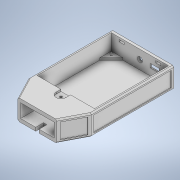
# Autodesk Inventor part: Bottom
Saved by Autodesk Inventor 2021 (Build 250183000, 183)
## iProperties
Created: 2021-04-28
Part Number: Bottom
Material: Generic
Document SubType Name: Modeling
Designer: mista
Density: 1 g/cm^3
Appearance: Default
Author: mista
Autodesk Inventor part; units mm, degrees
ref_plane "YZ Plane" through (0, 0, 0) normal (1, 0, 0) x (0, 1, 0)
ref_plane "XZ Plane" through (0, 0, 0) normal (0, 1, 0) x (-1, 0, 0)
ref_plane "XY Plane" through (0, 0, 0) normal (0, 0, 1) x (1, 0, 0)
sketch "Sketch1" plane through (0, 0, 0) normal (0, 1, 0) x (-1, 0, 0)
  line L0 (0, 0) -> (54.0004, 0)
  line L1 (54.0004, 0) -> (54.0004, -70.6374)
  line L2 (54.0004, -70.6374) -> (0, -70.6374)
  line L3 (0, -70.6374) -> (0, 0)
  circle A0 centre (51.9049, -68.5419) radius 1.0795
  circle A1 centre (3.3909, -67.8053) radius 1.0795
  circle A2 centre (51.9049, -1.8923) radius 1.0795
  circle A3 centre (1.7674, -2.3495) radius 1.0795
  dimension "d0" = 54.0004
  dimension "d1" = 70.6374
  dimension "d2" = 2.159
  dimension "d6" = 1.016
  dimension "d8" = 1.016
  dimension "d11" = 2.159
  dimension "d12" = 48.514
  dimension "d13" = 1.7526
  dimension "d15" = 66.6496
  dimension "d16" = 2.159
  dimension "d17" = 1.016
  dimension "d18" = 2.159
  dimension "d20" = 65.4558
  dimension "d21" = 50.1375
  constraints: 8 end point, 4 centre point, 2 parallel, 1 horizontal, 1 perpendicular
  measures "d0" distance of L1.end L2.end
  measures "d1" distance of L0.end L1.end
  measures "d2" diameter of A0
  measures "d6" distance edge to line of A0 L2
  measures "d8" distance edge to line of A0 L1
  measures "d11" diameter of A1
  measures "d12" horizontal distance of A1.centre A0.centre
  measures "d13" distance edge to line of A1 L2
  measures "d15" distance of A0.centre A2.centre
  measures "d16" diameter of A2
  measures "d17" distance edge to line of A2 L1
  measures "d18" diameter of A3
  measures "d20" vertical distance of A1.centre A3.centre
  measures "d21" horizontal distance of A3.centre A2.centre
sketch "Sketch2" plane through (0, 0, 0) normal (0, 1, 0) x (-1, 0, 0)
  line L0 (54.0004, 0) -> (54.0004, -70.6374) projected
  line L1 (0, 0) -> (54.0004, 0) projected
  line L2 (0, -70.6374) -> (0, 0) projected
  line L3 (54.0004, -70.6374) -> (0, -70.6374) projected
  line L4 (55.2704, -71.9074) -> (55.2704, 1.27)
  line L5 (55.2704, 1.27) -> (-1.27, 1.27)
  line L6 (-1.27, 1.27) -> (-1.27, -71.9074)
  line L7 (-1.27, -71.9074) -> (55.2704, -71.9074)
  line L8 (57.8104, 3.81) -> (57.8104, -74.4474)
  line L9 (57.8104, -74.4474) -> (-3.81, -74.4474)
  line L10 (-3.81, -74.4474) -> (-3.81, 3.81)
  line L11 (-3.81, 3.81) -> (57.8104, 3.81)
  dimension "d22" = 1.27
  dimension "d23" = 2.54
  constraints: 16 end point, 6 other
  measures "d22" distance between parallel lines of L0 L4
  measures "d23" distance between parallel lines of L4 L8
extrude "Extrusion1" add sketch "Sketch2" against normal blind 2.54 contours L0 L3 L2 L1 | L7 L6 L5 L4 | L8 L9 L10 L11
extrude "Extrusion2" add sketch "Sketch2" along normal blind 15.24 contours L8 L9 L10 L11
sketch "Sketch3" plane through (0, 0, 0) normal (0, 1, 0) x (1, 0, 0)
  line L0 (-55.2704, 71.9074) -> (-55.2704, -1.27) projected
  line L1 (-55.2704, -1.27) -> (1.27, -1.27) projected
  line L2 (1.27, -1.27) -> (1.27, 71.9074) projected
  line L3 (1.27, 71.9074) -> (-55.2704, 71.9074) projected
  line L4 (1.27, 10.16) -> (-10.16, -1.27)
  line L5 (-0.6357, 8.2543) -> (6.4192, 8.2543) construction
  line L6 (1.27, -1.27) -> (-55.2704, -1.27) construction
  line L7 (-27.0002, -1.27) -> (-27.0002, 8.9046) construction
  line L8 (1.27, 71.9074) -> (1.27, -1.27) construction
  line L9 (1.27, 35.3187) -> (-18.2366, 35.3187) construction
  line L10 (-55.2704, 10.16) -> (-43.8404, -1.27)
  line L11 (1.27, 60.4774) -> (-10.16, 71.9074)
  line L12 (-55.2704, 60.4774) -> (-43.8404, 71.9074)
  point P0 (0, 0)
  point P1 (-10.16, 71.9074)
  point P2 (1.27, 60.4774)
  point P3 (-55.2704, 60.4774)
  point P4 (-43.8404, 71.9074)
  dimension "d28" = 135
  dimension "d29" = 11.43
  constraints: 14 end point, 6 symmetric about line, 3 point on line, 2 horizontal, 2 midpoint, 1 vertical
  measures "d28" angle of L4 L5
  measures "d29" horizontal distance of L4.start L4.end
extrude "Extrusion3" add sketch "Sketch3" along normal blind 2.032 contours L3 L12 L0 | L10 L1 L0 | L3 L2 L11 | L4 L2 L1
extrude "Extrusion4" add sketch "Sketch1" along normal blind 3.81 contours A0 | A1 | A2 | A3
thicken "Thicken1" operation add thickness 0.127 both sides no extend neighbours yes toward (0.8451901, 0, -0.5344658) faces at (-4.3033, 3.2173, -67.2283)
thicken "Thicken2" operation add thickness 0.127 both sides no extend neighbours yes toward (0.9870503, 0, -0.1604113) faces at (-2.8329, 3.2173, -2.1763)
thicken "Thicken3" operation add thickness 0.127 both sides no extend neighbours yes toward (-0.6324454, 0, -0.774605) faces at (-51.2222, 3.2173, -1.0561)
thicken "Thicken4" operation add thickness 0.127 both sides no extend neighbours yes toward (-0.8451901, 0, 0.5344658) faces at (-50.9925, 2.6247, -69.1189)
sketch "Sketch10" plane through (3.81, -2.54, -74.4474) normal (0, 0, -1) x (-1, 0, 0)
  line L0 (20.6248, 13.4112) -> (20.6248, 9.6012)
  line L1 (20.6248, 9.6012) -> (11.7348, 9.6012)
  line L2 (11.7348, 9.6012) -> (11.7348, 13.4112)
  line L3 (11.7348, 13.4112) -> (20.6248, 13.4112)
  line L4 (0, 0) -> (0, 17.78)
  line L5 (61.6204, 0) -> (0, 0)
  line L6 (61.6204, 17.78) -> (61.6204, 0)
  line L7 (0, 17.78) -> (61.6204, 17.78)
  line L8 (22.1488, 13.9192) -> (22.1488, 9.0932)
  line L9 (21.1328, 8.0772) -> (11.2268, 8.0772)
  line L10 (10.2108, 9.0932) -> (10.2108, 13.9192)
  line L11 (11.2268, 14.9352) -> (21.1328, 14.9352)
  arc A0 (11.2268, 14.9352) -> (10.2108, 13.9192) centre (11.2268, 13.9192) ccw
  arc A1 (22.1488, 13.9192) -> (21.1328, 14.9352) centre (21.1328, 13.9192) ccw
  arc A2 (21.1328, 8.0772) -> (22.1488, 9.0932) centre (21.1328, 9.0932) ccw
  arc A3 (10.2108, 9.0932) -> (11.2268, 8.0772) centre (11.2268, 9.0932) ccw
  point P0 (3.81, 2.54)
  point P1 (57.8104, 2.54)
  dimension "d93" = 6.858
  dimension "d94" = 1.016
  constraints: 24 end point, 8 point on circle, 8 tangent, 4 centre point, 3 equal radius, 3 other
  measures "d93" distance between parallel lines of L9 L11
  measures "d94" radius of A0
extrude "Extrusion9" cut sketch "Sketch10" against normal blind 2.54 contours L0 L1 L2 L3
extrude "Extrusion10" cut sketch "Sketch10" against normal blind 1.27 contours L8 A2 L9 A3 L10 A0 L11 A1
sketch "Sketch11" plane through (3.81, -2.54, -74.4474) normal (0, 0, -1) x (-1, 0, 0)
  circle A0 centre (30.8102, 11.5062) radius 2.54 projected
  point P0 (3.81, 2.54)
extrude "Extrusion11" cut sketch "Sketch11" against normal blind 2.54
sketch "Sketch12" plane through (0, -2.54, 0) normal (0, -1, 0) x (1, 0, 0)
  line L0 (3.81, 3.81) -> (-57.8104, 3.81) projected
  line L1 (-57.8104, 3.81) -> (3.81, 3.81)
  line L2 (3.81, 3.81) -> (3.81, 29.21)
  line L3 (3.81, 29.21) -> (-57.8104, 29.21)
  line L4 (-57.8104, 29.21) -> (-57.8104, 3.81)
  point P0 (0, 0)
  dimension "d101" = 25.4
  constraints: 8 end point, 2 parallel, 1 horizontal, 1 perpendicular
  measures "d101" distance of L2.end L1.end
extrude "Extrusion12" add sketch "Sketch12" against normal up to surface (17.78 mm away)
sketch "Sketch14" plane through (0, 15.24, 0) normal (0, 1, 0) x (1, 0, 0)
  line L0 (3.81, 74.4474) -> (3.81, -29.21) projected
  line L1 (3.81, 74.4474) -> (-57.8104, 74.4474) projected
  line L2 (-57.8104, 74.4474) -> (-57.8104, -29.21) projected
  line L3 (3.81, -29.21) -> (-57.8104, -29.21) projected
  line L4 (-55.2704, 71.9074) -> (1.27, 71.9074) projected
  line L5 (1.27, 71.9074) -> (1.27, -1.27) projected
  line L6 (1.27, -1.27) -> (-55.2704, -1.27) projected
  line L7 (-55.2704, -1.27) -> (-55.2704, 71.9074) projected
  point P0 (0, 0)
extrude "Extrusion13" add sketch "Sketch14" along normal blind 2.54
sketch "Sketch15" plane through (-57.8104, -2.54, 29.21) normal (0, 0, 1) x (1, 0, 0)
  line L0 (14.1732, 16.891) -> (47.4472, 16.891)
  line L1 (47.4472, 16.891) -> (47.4472, 3.429)
  line L2 (47.4472, 3.429) -> (14.1732, 3.429)
  line L3 (14.1732, 3.429) -> (14.1732, 16.891)
  line L4 (14.1732, 10.16) -> (47.4472, 10.16) construction
  line L5 (30.8102, 16.891) -> (30.8102, 3.429) construction
  line L6 (0, 0) -> (0, 20.32) construction
  line L7 (0, 10.16) -> (62.1543, 10.16) construction
  line L8 (0, 0) -> (61.6204, 0) construction
  line L9 (30.8102, 0) -> (30.8102, 10.16) construction
  point P0 (57.8104, 2.54)
  point P1 (57.8104, 2.54)
  dimension "d108" = 13.462
  dimension "d109" = 33.274
  dimension "d110" = 0
  dimension "d112" = 0
  constraints: 16 end point, 6 midpoint, 2 horizontal, 2 parallel, 2 perpendicular, 1 point on line
  measures "d108" distance of L0.end L1.end
  measures "d109" distance of L0.start L0.end
  measures "d110" distance between parallel lines of L7 L4
  measures "d112" distance between parallel lines of L9 L5
extrude "Extrusion14" cut sketch "Sketch15" against normal blind 14.2748
sketch "Sketch17" plane through (-10.16, 0, 1.27) normal (0, 0, -1) x (-1, 0, 0)
  line L0 (0.2032, 0.889) -> (33.4772, 0.889) projected
  line L1 (0.2032, 14.351) -> (0.2032, 0.889) projected
  line L2 (33.4772, 14.351) -> (0.2032, 14.351) projected
  line L3 (33.4772, 0.889) -> (33.4772, 14.351) projected
  line L4 (-11.43, 2.032) -> (0, 2.032) projected
  line L5 (33.6804, 2.032) -> (45.1104, 2.032) projected
  line L6 (-2.3368, 5.842) -> (36.0172, 5.842)
  line L7 (-2.3368, 0.889) -> (-2.3368, 2.032)
  line L8 (-2.3368, 5.842) -> (-2.3368, 15.4602)
  line L9 (36.0172, 15.4602) -> (36.0172, 5.842)
  line L10 (36.0172, 2.032) -> (36.0172, 0.889)
  line L11 (0.2032, 14.351) -> (-2.3368, 14.351)
  line L12 (0.2032, 14.351) -> (36.0172, 14.351)
  point P0 (-10.16, 0)
  constraints: 14 end point, 5 point on line, 1 perpendicular
loft "Loft1" cut profiles "Sketch17" section 2 edges at (-27.0002, 0.889, 14.9352) (-10.3632, 7.62, 14.9352) (-27.0002, 14.351, 14.9352) (-43.6372, 7.62, 14.9352) contours L6 L8 L11 L1 | L1 L2 L3 L6 | L3 L12 L9 L6
sketch "Sketch20" plane through (0, 17.78, 0) normal (0, 1, 0) x (1, 0, 0)
  line L0 (-43.6372, -29.21) -> (-10.3632, -29.21) projected
  line L1 (-10.3632, -29.21) -> (-43.6372, -29.21) projected
  line L2 (1.27, -1.27) -> (-55.2704, -1.27) projected
  line L3 (3.81, -6.8796) -> (-57.8104, -6.8796)
  line L4 (-57.8104, 74.4474) -> (-57.8104, -29.21) projected
  line L5 (3.81, -29.21) -> (3.81, 74.4474) projected
  line L6 (-43.6372, -29.21) -> (-43.6372, -14.9352) projected
  line L7 (-43.6372, -29.21) -> (-46.1772, -29.21)
  line L8 (-57.8104, -29.21) -> (3.81, -29.21) projected
  line L9 (-46.1772, -29.21) -> (-57.8104, -6.8796)
  line L10 (-10.3632, -29.21) -> (-10.3632, -14.9352) projected
  line L11 (-10.3632, -29.21) -> (-7.8232, -29.21)
  line L12 (-7.8232, -29.21) -> (3.81, -6.8796)
  line L13 (-57.8104, -29.21) -> (-46.1772, -29.21)
  line L14 (-57.8104, -29.21) -> (-57.8104, -6.8796)
  line L15 (-7.8232, -29.21) -> (3.81, -29.21)
  line L16 (3.81, -6.8796) -> (3.81, -29.21)
  point P0 (0, 0)
  dimension "d123" = 2.54
  dimension "d124" = 2.54
  constraints: 18 end point, 4 point on line, 2 collinear, 2 perpendicular, 1 parallel
  measures "d123" distance of L0.start L7.end
  measures "d124" distance of L0.end L11.end
extrude "Extrusion15" cut sketch "Sketch20" against normal through all contours L8 L4 L9 | L12 L5 L8
sketch "Sketch22" plane through (0, 17.78, 0) normal (0, 1, 0) x (1, 0, 0)
  line L0 (-55.2704, 71.9074) -> (1.27, 71.9074) projected
  line L1 (1.27, 71.9074) -> (1.27, -1.27) projected
  line L2 (1.27, -1.27) -> (-55.2704, -1.27) projected
  line L3 (-55.2704, -1.27) -> (-55.2704, 71.9074) projected
  line L4 (-7.8232, -29.21) -> (3.81, -6.8796) projected
  line L5 (3.81, -6.8796) -> (3.81, 74.4474) projected
  line L6 (3.81, 74.4474) -> (-57.8104, 74.4474) projected
  line L7 (-57.8104, 74.4474) -> (-57.8104, -6.8796) projected
  line L8 (-57.8104, -6.8796) -> (-46.1772, -29.21) projected
  line L9 (-46.1772, -29.21) -> (-7.8232, -29.21) projected
  line L10 (-43.8404, -1.27) -> (-10.16, -1.27) construction
  line L11 (-27.0002, -1.27) -> (-27.0002, -14.9352) construction
  line L12 (-10.3632, -14.9352) -> (-43.6372, -14.9352) construction
  circle A0 centre (-27.0002, -6.0325) radius 4.7625
  line L13 (-22.2377, -6.0325) -> (-22.2377, -1.27)
  line L14 (-31.7627, -6.0325) -> (-31.7627, -1.27)
  point P0 (0, 0)
  dimension "d127" = 9.525
  dimension "d128" = 4.7625
  constraints: 6 end point, 3 point on line, 2 midpoint, 2 perpendicular, 2 point on circle, 1 centre point, 1 tangent
  measures "d127" diameter of A0
  measures "d128" distance from line of L2 A0.centre
extrude "Extrusion16" cut sketch "Sketch22" against normal blind 1.778 contours L2 A0 L14 | L13 A0 L2 | A0
sketch "Sketch23" plane through (-43.8404, 0, -71.9074) normal (0, 0, 1) x (1, 0, 0)
  circle A0 centre (16.8402, 8.9662) radius 2.54 projected
  line L0 (27.0256, 10.8712) -> (35.9156, 10.8712) projected
  line L1 (35.9156, 10.8712) -> (35.9156, 7.0612) projected
  line L2 (35.9156, 7.0612) -> (27.0256, 7.0612) projected
  line L3 (27.0256, 7.0612) -> (27.0256, 10.8712) projected
  line L4 (33.6804, 0) -> (33.6804, 2.032) projected
  line L5 (33.6804, 2.032) -> (45.1104, 2.032) projected
  line L6 (45.1104, 2.032) -> (45.1104, 17.78) projected
  line L7 (-11.43, 17.78) -> (45.1104, 17.78) projected
  line L8 (-11.43, 2.032) -> (-11.43, 17.78) projected
  line L9 (-11.43, 2.032) -> (0, 2.032) projected
  line L10 (0, 2.032) -> (0, 0) projected
  line L11 (33.6804, 0) -> (0, 0) projected
  line L12 (-3.81, 15.875) -> (1.27, 15.875)
  line L13 (1.27, 15.875) -> (1.27, 13.97)
  line L14 (1.27, 13.97) -> (-3.81, 13.97)
  line L15 (-3.81, 13.97) -> (-3.81, 15.875)
  line L16 (-11.43, 17.78) -> (45.1104, 17.78) construction
  line L17 (16.8402, 17.78) -> (16.8402, 15.24) construction
  line L18 (37.4904, 15.875) -> (32.4104, 15.875)
  line L19 (32.4104, 15.875) -> (32.4104, 13.97)
  line L20 (32.4104, 13.97) -> (37.4904, 13.97)
  line L21 (37.4904, 13.97) -> (37.4904, 15.875)
  point P0 (43.8404, 0)
  dimension "d131" = 1.905
  dimension "d132" = 5.08
  dimension "d133" = 1.905
  dimension "d134" = 7.62
  constraints: 18 end point, 4 symmetric about line, 2 parallel, 1 horizontal, 1 midpoint, 1 perpendicular, 1 vertical
  measures "d131" distance of L14.end L12.start
  measures "d132" distance of L13.end L14.end
  measures "d133" distance between parallel lines of L12 L7
  measures "d134" distance between parallel lines of L8 L15
extrude "Extrusion17" cut sketch "Sketch23" against normal through all contours L12 L13 L14 L15 | L21 L20 L19 L18
sketch "Sketch26" plane through (0, 16.002, 0) normal (0, 1, 0) x (1, 0, 0)
  line L0 (-22.2377, -1.27) -> (-22.2377, -6.0325) projected
  line L1 (-31.7627, -1.27) -> (-22.2377, -1.27) projected
  line L2 (-31.7627, -6.0325) -> (-31.7627, -1.27) projected
  arc A0 (-31.7627, -6.0325) -> (-22.2377, -6.0325) centre (-27.0002, -6.0325) ccw projected
  circle A1 centre (-27.0002, -6.0325) radius 1.143
  point P0 (0, 0)
  dimension "d137" = 2.286
  constraints: 1 centre point, 1 coincident
  measures "d137" diameter of A1
extrude "Extrusion18" cut sketch "Sketch26" against normal up to next contours A1
sketch "Sketch27" plane through (0, 17.78, 0) normal (0, 1, 0) x (1, 0, 0)
  circle A0 centre (-27.0002, -6.0325) radius 1.143 projected
  line L0 (-22.2377, -1.27) -> (-22.2377, -6.0325) projected
  line L1 (-31.7627, -1.27) -> (-22.2377, -1.27) projected
  line L2 (-31.7627, -6.0325) -> (-31.7627, -1.27) projected
  arc A1 (-31.7627, -6.0325) -> (-22.2377, -6.0325) centre (-27.0002, -6.0325) ccw projected
  line L3 (-7.8232, -29.21) -> (3.81, -6.8796) projected
  line L4 (3.81, -6.8796) -> (3.81, 74.4474) projected
  line L5 (3.81, 74.4474) -> (-57.8104, 74.4474) projected
  line L6 (-57.8104, 74.4474) -> (-57.8104, -6.8796) projected
  line L7 (-57.8104, -6.8796) -> (-46.1772, -29.21) projected
  line L8 (-46.1772, -29.21) -> (-7.8232, -29.21) projected
  line L9 (-22.2377, -1.27) -> (-22.2377, -6.0325) projected
  arc A2 (-31.7627, -6.0325) -> (-22.2377, -6.0325) centre (-27.0002, -6.0325) ccw projected
  line L10 (-31.7627, -6.0325) -> (-31.7627, -1.27) projected
  line L11 (-31.7627, -1.27) -> (-55.2704, -1.27) projected
  line L12 (-55.2704, -1.27) -> (-55.2704, 71.9074) projected
  line L13 (-55.2704, 71.9074) -> (1.27, 71.9074) projected
  line L14 (1.27, 71.9074) -> (1.27, -1.27) projected
  line L15 (1.27, -1.27) -> (-22.2377, -1.27) projected
  line L16 (-11.43, 74.4474) -> (-6.35, 74.4474) projected
  line L17 (-11.43, 71.9074) -> (-11.43, 74.4474) projected
  line L18 (-6.35, 71.9074) -> (-11.43, 71.9074) projected
  line L19 (-6.35, 71.9074) -> (-6.35, 74.4474) projected
  line L20 (-47.6504, 74.4474) -> (-42.5704, 74.4474) projected
  line L21 (-47.6504, 71.9074) -> (-47.6504, 74.4474) projected
  line L22 (-42.5704, 71.9074) -> (-47.6504, 71.9074) projected
  line L23 (-42.5704, 71.9074) -> (-42.5704, 74.4474) projected
  point P0 (0, 0)
sketch "Sketch28" plane through (0, -2.54, 0) normal (0, -1, 0) x (1, 0, 0)
  line L0 (-7.8232, 29.21) -> (-46.1772, 29.21) construction
  line L1 (-27.0002, 29.21) -> (-27.0002, 17.9289) construction
  line L2 (-28.6512, 29.21) -> (-28.6512, 21.59)
  line L3 (-25.3492, 29.21) -> (-25.3492, 21.59)
  line L4 (-25.3492, 21.59) -> (-28.6512, 21.59)
  line L5 (-28.6512, 29.21) -> (-25.3492, 29.21)
  point P0 (0, 0)
  dimension "d140" = 1.651
  dimension "d141" = 1.651
  dimension "d142" = 7.62
  dimension "d143" = 0
  constraints: 10 end point, 3 parallel, 1 midpoint, 1 perpendicular, 1 vertical
  measures "d140" distance between parallel lines of L1 L2
  measures "d141" distance between parallel lines of L1 L3
  measures "d142" distance of L3.start L3.end
  measures "d143" distance from line of L0 L3.start
extrude "Extrusion19" cut sketch "Sketch28" against normal up to next
sketch "Sketch29" plane through (3.81, -2.54, -74.4474) normal (1, 0, 0) x (0, 0, -1)
  line L0 (-81.327, 20.32) -> (-81.327, 0) projected
  line L1 (0, 0) -> (-81.327, 0) projected
  line L2 (0, 0) -> (0, 20.32) projected
  line L3 (-81.327, 20.32) -> (0, 20.32) projected
  line L4 (-2.54, 17.78) -> (-2.54, 2.54)
  line L5 (-2.54, 2.54) -> (-78.787, 2.54)
  line L6 (-78.787, 2.54) -> (-78.787, 17.78)
  line L7 (-78.787, 17.78) -> (-2.54, 17.78)
  point P0 (-74.4474, 2.54)
  dimension "d146" = 2.54
  constraints: 8 end point, 3 other
  measures "d146" distance between parallel lines of L3 L7
extrude "Extrusion20" cut sketch "Sketch29" against normal blind 0.762 contours L4 L5 L6 L7
sketch "Sketch30" plane through (3.81, -2.54, 6.8796) normal (0.8868688, 0, 0.4620214) x (0.4620214, 0, -0.8868688)
  line L0 (0, 0) -> (-25.1789, 0) projected
  line L1 (0, 20.32) -> (0, 0) projected
  line L2 (-25.1789, 20.32) -> (0, 20.32) projected
  line L3 (-25.1789, 0) -> (-25.1789, 20.32) projected
  line L4 (-2.54, 17.78) -> (-2.54, 2.54)
  line L5 (-2.54, 2.54) -> (-22.6389, 2.54)
  line L6 (-22.6389, 2.54) -> (-22.6389, 17.78)
  line L7 (-22.6389, 17.78) -> (-2.54, 17.78)
  point P0 (4.341, 2.54)
  dimension "d149" = 2.54
  constraints: 8 end point, 3 other
  measures "d149" distance between parallel lines of L2 L7
extrude "Extrusion21" cut sketch "Sketch30" against normal blind 0.762 contours L4 L5 L6 L7
sketch "Sketch31" plane through (-46.1772, -2.54, 29.21) normal (-0.8868688, 0, 0.4620214) x (0.4620214, 0, 0.8868688)
  line L0 (0, 0) -> (-25.1789, 0) projected
  line L1 (0, 20.32) -> (0, 0) projected
  line L2 (-25.1789, 20.32) -> (0, 20.32) projected
  line L3 (-25.1789, 0) -> (-25.1789, 20.32) projected
  line L4 (-2.54, 17.78) -> (-2.54, 2.54)
  line L5 (-2.54, 2.54) -> (-22.6389, 2.54)
  line L6 (-22.6389, 2.54) -> (-22.6389, 17.78)
  line L7 (-22.6389, 17.78) -> (-2.54, 17.78)
  point P0 (-4.5706, 2.54)
  dimension "d152" = 2.54
  constraints: 8 end point, 3 other
  measures "d152" distance between parallel lines of L2 L7
extrude "Extrusion22" cut sketch "Sketch31" against normal blind 0.762 contours L4 L5 L6 L7
sketch "Sketch32" plane through (-57.8104, -2.54, -74.4474) normal (-1, 0, 0) x (0, 0, 1)
  line L0 (81.327, 0) -> (81.327, 20.32) projected
  line L1 (0, 20.32) -> (81.327, 20.32) projected
  line L2 (0, 0) -> (0, 20.32) projected
  line L3 (81.327, 0) -> (0, 0) projected
  line L4 (78.787, 17.78) -> (78.787, 2.54)
  line L5 (78.787, 2.54) -> (2.54, 2.54)
  line L6 (2.54, 2.54) -> (2.54, 17.78)
  line L7 (2.54, 17.78) -> (78.787, 17.78)
  point P0 (74.4474, 2.54)
  dimension "d155" = 2.54
  constraints: 8 end point, 3 other
  measures "d155" distance between parallel lines of L1 L7
extrude "Extrusion23" cut sketch "Sketch32" against normal blind 0.762 contours L4 L5 L6 L7
chamfer "Chamfer1" distance 1.27 angle 45 8 edges at (-2.0066, 17.78, 18.0448) (3.81, 17.78, -33.7839) (-57.8104, 17.78, -33.7839) (-51.9938, 17.78, 18.0448) (3.81, -2.54, -33.7839) (-2.0066, -2.54, 18.0448) (-57.8104, -2.54, -33.7839) (-51.9938, -2.54, 18.0448)
sketch "Sketch33" plane through (0, -2.54, 0) normal (0, -1, 0) x (1, 0, 0)
  line L0 (-56.5404, 6.5686) -> (-44.7452, 29.21) projected
  line L1 (-56.5404, -74.4474) -> (-56.5404, 6.5686) projected
  line L2 (-56.5404, -74.4474) -> (2.54, -74.4474) projected
  line L3 (2.54, 6.5686) -> (2.54, -74.4474) projected
  line L4 (-9.2552, 29.21) -> (2.54, 6.5686) projected
  line L5 (-9.2552, 29.21) -> (-25.3492, 29.21) projected
  line L6 (-25.3492, 29.21) -> (-25.3492, 21.59) projected
  line L7 (-25.3492, 21.59) -> (-28.6512, 21.59) projected
  line L8 (-28.6512, 21.59) -> (-28.6512, 29.21) projected
  line L9 (-28.6512, 29.21) -> (-44.7452, 29.21) projected
  line L10 (-5.08, 4.7028) -> (-5.08, -66.8274)
  line L11 (-5.08, -66.8274) -> (-48.9204, -66.8274)
  line L12 (-48.9204, -66.8274) -> (-48.9204, 4.7028)
  line L13 (-48.9204, 4.7028) -> (-44.0926, 13.97)
  line L14 (-44.0926, 13.97) -> (-9.9078, 13.97)
  line L15 (-9.9078, 13.97) -> (-5.08, 4.7028)
  point P0 (0, 0)
  dimension "d161" = 7.62
  constraints: 12 end point, 2 other
  measures "d161" distance between parallel lines of L4 L15
extrude "Extrusion24" cut sketch "Sketch33" against normal blind 0.762 contours L10 L11 L12 L13 L14 L15
body "Solid1"
